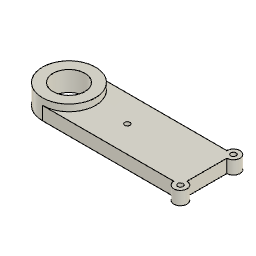
encoder-holder (Autodesk Fusion 360 design; units mm, degrees)
Autodesk Fusion 360 part; units mm, degrees
note: some values were not read from the file. Set by a fixed rule: which sketch regions a step uses.
sketch "Skizze1" plane through (0, 0, 0) normal (0, 0, 1) x (1, 0, 0)
  circle A0 centre (0, 0) radius 6
  circle A1 centre (0, 0) radius 10
  line L0 (0, 0) -> (22, 0) construction
  circle A2 centre (22, 0) radius 1
  line L1 (22, 0) -> (52, 0) construction
  line L2 (52, 0) -> (52, 10) construction
  line L3 (52, 0) -> (52, -10) construction
  circle A3 centre (52, 10) radius 1
  circle A4 centre (52, -10) radius 1
  line L4 (0, 10) -> (52, 10)
  line L5 (52, 10) -> (52, -10)
  line L6 (52, -10) -> (0, -10)
  line L7 (0, -10) -> (0, 10)
  circle A5 centre (52, 10) radius 2.5
  circle A6 centre (52, -10) radius 2.5
  dimension "d1" = 12
  dimension "d2" = 20
  dimension "d3" = 22
  dimension "d4" = 2
  dimension "d5" = 30
  dimension "d6" = 10
  dimension "d7" = 10
  dimension "d8" = 2
  dimension "d9" = 2
  dimension "d10" = 5
  dimension "d11" = 5
  constraint coincident A0.centre A1.centre
  constraint concentric A0 A1
  constraint horizontal L0
  constraint coincident L0.end A2.centre
  constraint parallel L0 L1
  constraint perpendicular L1 L2
  constraint perpendicular L1 L3
  constraint coincident L2.end A3.centre
  constraint coincident L3.end A4.centre
  constraint horizontal L4
  constraint vertical L5
  constraint horizontal L6
  constraint vertical L7
  constraint coincident A1 L4.start
  measures "d1" diameter of A0
  measures "d2" diameter of A1
  measures "d3" distance of A0.centre L0.end
  measures "d4" diameter of A2
  measures "d5" distance of L0.end L1.end
  measures "d6" distance of L1.end L2.end
  measures "d7" distance of L1.end L3.end
  measures "d8" diameter of A3
  measures "d9" diameter of A4
  measures "d10" diameter of A5
  measures "d11" diameter of A6
extrude "Extrusion1" add sketch "Skizze1" along normal blind 5 contours A0 A1 L7 | A0 A1 L7 | A1 L4 L5 L6 A5 A6 | A3 L4 L5 A5 | A3 L4 L5 A5 | A4 L5 L6 A6 | A4 L5 L6 A6
sketch "Skizze2" plane through (0, 0, 5) normal (0, 0, 1) x (-1, 0, 0)
  circle A0 centre (0, 0) radius 6
  circle A1 centre (-52, -10) radius 1
  circle A2 centre (-52, 10) radius 1
  circle A3 centre (-22, 0) radius 1
  arc A4 (0, -10) -> (0, 10) centre (0, 0) ccw
  line L0 (0, 10) -> (-49.5, 10)
  arc A5 (-49.5, 10) -> (-52, 7.5) centre (-52, 10) ccw
  line L1 (-52, 7.5) -> (-52, -7.5)
  arc A6 (-52, -7.5) -> (-49.5, -10) centre (-52, -10) ccw
  line L2 (-49.5, -10) -> (0, -10)
  circle A7 centre (0, 0) radius 10
  constraint concentric A0 A7
extrude "Extrusion2" add sketch "Skizze2" along normal blind 2.5 contours A4 A7
